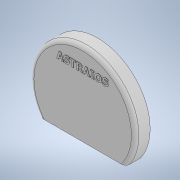
# Autodesk Inventor part: SensorCap_v2
Saved by Autodesk Inventor 2020 (Build 240168000, 168)
## iProperties
Created: 2020-03-11
Part Number: SensorCap_v2
Material: Generic
Document SubType Name: Modeling
Designer: WANG
Density: 1 g/cm^3
Appearance: Default
Author: WANG
Autodesk Inventor part; units mm, degrees
ref_plane "YZ Plane" through (0, 0, 0) normal (1, 0, 0) x (0, 1, 0)
ref_plane "XZ Plane" through (0, 0, 0) normal (0, 1, 0) x (-1, 0, 0)
ref_plane "XY Plane" through (0, 0, 0) normal (0, 0, 1) x (1, 0, 0)
sketch "Sketch1" plane through (0, 0, 0) normal (0, 0, 1) x (1, 0, 0)
  circle A0 centre (0, 0) radius 44.45
  circle A1 centre (0, 0) radius 41.275
  dimension "d0" = 88.9
  dimension "d1" = 82.55
  constraints: 2 centre point, 2 coincident
  measures "d0" diameter of A0
  measures "d1" diameter of A1
extrude "Extrusion1" add sketch "Sketch1" along normal blind 12.7 contours A0 | A1
sketch "Sketch2" plane through (0, 0, 0) normal (0, 0, -1) x (-1, 0, 0)
  circle A0 centre (0, 0) radius 44.45
  circle A1 centre (0, 0) radius 41.275
  dimension "d4" = 88.9
  dimension "d5" = 82.55
  constraints: 2 centre point, 2 coincident
  measures "d4" diameter of A0
  measures "d5" diameter of A1
extrude "Extrusion2" cut sketch "Sketch2" against normal blind 9.525 contours A1
sketch "Sketch3" plane through (0, 0, 12.7) normal (0, 0, 1) x (1, 0, 0)
  circle A0 centre (0, 0) radius 44.45
  line L0 (0, -25.4) -> (36.478, -25.4)
  line L1 (0, -25.4) -> (-36.478, -25.4)
  circle A1 centre (0, 0) radius 44.45 projected
  dimension "d8" = 88.9
  dimension "d9" = 25.4
  constraints: 4 end point, 1 coincident, 1 horizontal, 1 point on circle, 1 point on line, 3 other
  measures "d9" distance of L0.start point (0, 0)
extrude "Extrusion3" cut sketch "Sketch3" against normal up to surface (12.7 mm away) contours L1 L0 A0 picked at (-22.4742, -27.57)
fillet "Fillet1" radius 3.175 1 edges at (0, 44.45, 12.7)
sketch "Sketch4" plane through (0, 0, 12.7) normal (0, 0, 1) x (1, 0, 0)
  line L0 (-21.9003, 31.3927) -> (21.9277, 31.3927) construction
  line L1 (21.9277, 31.3927) -> (21.9277, 25.0398) construction
  line L2 (21.9277, 25.0398) -> (-21.9003, 25.0398) construction
  line L3 (-21.9003, 25.0398) -> (-21.9003, 31.3927) construction
  line L4 (-21.925, 25.1683) -> (-19.865, 31.2643)
  line L5 (-19.865, 31.2643) -> (-18.1953, 31.2643)
  line L6 (-18.1953, 31.2643) -> (-16.1353, 25.1683)
  line L7 (-16.1353, 25.1683) -> (-17.7112, 25.1683)
  line L8 (-17.7112, 25.1683) -> (-18.0915, 26.4132)
  line L9 (-18.0915, 26.4132) -> (-20.0083, 26.4132)
  line L10 (-20.0083, 26.4132) -> (-20.3936, 25.1683)
  line L11 (-20.3936, 25.1683) -> (-21.925, 25.1683)
  line L12 (-18.4275, 27.5197) -> (-19.0499, 29.5353)
  line L13 (-19.0499, 29.5353) -> (-19.6773, 27.5197)
  line L14 (-19.6773, 27.5197) -> (-18.4275, 27.5197)
  spline S0 degree 2 poles (-13.6455, 25.0596) (-14.347, 25.0596) (-15.4042, 25.3313) (-15.8587, 25.5289) knots 0 0 0 1 2 2 2
  line L15 (-15.8587, 25.5289) -> (-15.8587, 26.9813)
  line L16 (-15.8587, 26.9813) -> (-15.7203, 26.9813)
  spline S1 degree 2 poles (-15.7203, 26.9813) (-15.2609, 26.591) (-14.1593, 26.1711) (-13.6406, 26.1711) knots 0 0 0 1 2 2 2
  spline S2 degree 2 poles (-13.6406, 26.1711) (-13.5072, 26.1711) (-13.0774, 26.2304) (-12.949, 26.2897) knots 0 0 0 1 2 2 2
  spline S3 degree 2 poles (-12.949, 26.2897) (-12.7909, 26.3588) (-12.5686, 26.6108) (-12.5686, 26.8133) knots 0 0 0 1 2 2 2
  spline S4 degree 2 poles (-12.5686, 26.8133) (-12.5686, 27.0455) (-12.9292, 27.332) (-13.1762, 27.3962) knots 0 0 0 1 2 2 2
  spline S5 degree 2 poles (-13.1762, 27.3962) (-13.4874, 27.4802) (-14.1939, 27.6235) (-14.5051, 27.7321) knots 0 0 0 1 2 2 2
  spline S6 degree 2 poles (-14.5051, 27.7321) (-15.2115, 27.9791) (-15.8241, 28.8239) (-15.8241, 29.4562) knots 0 0 0 1 2 2 2
  spline S7 degree 2 poles (-15.8241, 29.4562) (-15.8241, 30.3108) (-14.3766, 31.3729) (-13.2898, 31.3729) knots 0 0 0 1 2 2 2
  spline S8 degree 2 poles (-13.2898, 31.3729) (-12.7464, 31.3729) (-11.6695, 31.1506) (-11.2447, 30.9629) knots 0 0 0 1 2 2 2
  line L17 (-11.2447, 30.9629) -> (-11.2447, 29.5698)
  line L18 (-11.2447, 29.5698) -> (-11.378, 29.5698)
  spline S9 degree 2 poles (-11.378, 29.5698) (-11.7189, 29.8613) (-12.697, 30.2614) (-13.2108, 30.2614) knots 0 0 0 1 2 2 2
  spline S10 degree 2 poles (-13.2108, 30.2614) (-13.4133, 30.2614) (-13.7295, 30.2022) (-13.9073, 30.1231) knots 0 0 0 1 2 2 2
  spline S11 degree 2 poles (-13.9073, 30.1231) (-14.0506, 30.0589) (-14.2581, 29.802) (-14.2581, 29.6439) knots 0 0 0 1 2 2 2
  spline S12 degree 2 poles (-14.2581, 29.6439) (-14.2581, 29.4068) (-13.9271, 29.1351) (-13.4529, 29.0264) knots 0 0 0 1 2 2 2
  spline S13 degree 2 poles (-13.4529, 29.0264) (-13.1466, 28.9573) (-12.5785, 28.8239) (-12.2524, 28.7103) knots 0 0 0 1 2 2 2
  spline S14 degree 2 poles (-12.2524, 28.7103) (-11.6201, 28.4781) (-11.0026, 27.7074) (-11.0026, 27.0751) knots 0 0 0 1 2 2 2
  spline S15 degree 2 poles (-11.0026, 27.0751) (-11.0026, 26.1662) (-12.4303, 25.0596) (-13.6455, 25.0596) knots 0 0 0 1 2 2 2
  line L19 (-9.0463, 25.1683) -> (-9.0463, 30.1034)
  line L20 (-9.0463, 30.1034) -> (-10.8495, 30.1034)
  line L21 (-10.8495, 30.1034) -> (-10.8495, 31.2643)
  line L22 (-10.8495, 31.2643) -> (-5.7118, 31.2643)
  line L23 (-5.7118, 31.2643) -> (-5.7118, 30.1034)
  line L24 (-5.7118, 30.1034) -> (-7.5149, 30.1034)
  line L25 (-7.5149, 30.1034) -> (-7.5149, 25.1683)
  line L26 (-7.5149, 25.1683) -> (-9.0463, 25.1683)
  line L27 (0.5472, 25.1683) -> (-1.3152, 25.1683)
  line L28 (-1.3152, 25.1683) -> (-3.0096, 27.4061)
  line L29 (-3.0096, 27.4061) -> (-3.5629, 27.4061)
  line L30 (-3.5629, 27.4061) -> (-3.5629, 25.1683)
  line L31 (-3.5629, 25.1683) -> (-5.0844, 25.1683)
  line L32 (-5.0844, 25.1683) -> (-5.0844, 31.2643)
  line L33 (-5.0844, 31.2643) -> (-2.6342, 31.2643)
  spline S16 degree 2 poles (-2.6342, 31.2643) (-2.1254, 31.2643) (-1.3745, 31.1358) (-1.0534, 30.9382) knots 0 0 0 1 2 2 2
  spline S17 degree 2 poles (-1.0534, 30.9382) (-0.7273, 30.7307) (-0.342, 30.0836) (-0.342, 29.5896) knots 0 0 0 1 2 2 2
  spline S18 degree 2 poles (-0.342, 29.5896) (-0.342, 28.893) (-0.9743, 28.0187) (-1.5029, 27.7618) knots 0 0 0 1 2 2 2
  line L34 (-1.5029, 27.7618) -> (0.5472, 25.1683)
  spline S19 degree 2 poles (-1.9129, 29.3969) (-1.9129, 29.6291) (-2.0908, 29.9601) (-2.2933, 30.049) knots 0 0 0 1 2 2 2
  spline S20 degree 2 poles (-2.2933, 30.049) (-2.4366, 30.1083) (-2.7873, 30.1429) (-3.0491, 30.1429) knots 0 0 0 1 2 2 2
  line L35 (-3.0491, 30.1429) -> (-3.5629, 30.1429)
  line L36 (-3.5629, 30.1429) -> (-3.5629, 28.5028)
  line L37 (-3.5629, 28.5028) -> (-3.1232, 28.5028)
  spline S21 degree 2 poles (-3.1232, 28.5028) (-2.8071, 28.5028) (-2.3575, 28.5818) (-2.2044, 28.7053) knots 0 0 0 1 2 2 2
  spline S22 degree 2 poles (-2.2044, 28.7053) (-2.0562, 28.8239) (-1.9129, 29.1401) (-1.9129, 29.3969) knots 0 0 0 1 2 2 2
  line L38 (0.3447, 25.1683) -> (2.4046, 31.2643)
  line L39 (2.4046, 31.2643) -> (4.0744, 31.2643)
  line L40 (4.0744, 31.2643) -> (6.1344, 25.1683)
  line L41 (6.1344, 25.1683) -> (4.5585, 25.1683)
  line L42 (4.5585, 25.1683) -> (4.1781, 26.4132)
  line L43 (4.1781, 26.4132) -> (2.2614, 26.4132)
  line L44 (2.2614, 26.4132) -> (1.8761, 25.1683)
  line L45 (1.8761, 25.1683) -> (0.3447, 25.1683)
  line L46 (3.8422, 27.5197) -> (3.2198, 29.5353)
  line L47 (3.2198, 29.5353) -> (2.5924, 27.5197)
  line L48 (2.5924, 27.5197) -> (3.8422, 27.5197)
  line L49 (9.7752, 25.1683) -> (6.495, 25.1683)
  line L50 (6.495, 25.1683) -> (6.495, 26.2304)
  line L51 (6.495, 26.2304) -> (7.3694, 26.2304)
  line L52 (7.3694, 26.2304) -> (7.3694, 30.2022)
  line L53 (7.3694, 30.2022) -> (6.495, 30.2022)
  line L54 (6.495, 30.2022) -> (6.495, 31.2643)
  line L55 (6.495, 31.2643) -> (9.7752, 31.2643)
  line L56 (9.7752, 31.2643) -> (9.7752, 30.2022)
  line L57 (9.7752, 30.2022) -> (8.9008, 30.2022)
  line L58 (8.9008, 30.2022) -> (8.9008, 26.2304)
  line L59 (8.9008, 26.2304) -> (9.7752, 26.2304)
  line L60 (9.7752, 26.2304) -> (9.7752, 25.1683)
  spline S23 degree 2 poles (16.3405, 28.2163) (16.3405, 26.7343) (14.7597, 25.0398) (13.3863, 25.0398) knots 0 0 0 1 2 2 2
  spline S24 degree 2 poles (13.3863, 25.0398) (12.0081, 25.0398) (10.4371, 26.754) (10.4371, 28.2163) knots 0 0 0 1 2 2 2
  spline S25 degree 2 poles (10.4371, 28.2163) (10.4371, 29.6835) (12.0081, 31.3927) (13.3863, 31.3927) knots 0 0 0 1 2 2 2
  spline S26 degree 2 poles (13.3863, 31.3927) (14.7597, 31.3927) (16.3405, 29.6933) (16.3405, 28.2163) knots 0 0 0 1 2 2 2
  spline S27 degree 2 poles (14.7597, 28.2163) (14.7597, 28.7646) (14.5374, 29.5303) (14.3447, 29.7724) knots 0 0 0 1 2 2 2
  spline S28 degree 2 poles (14.3447, 29.7724) (14.152, 30.0243) (13.658, 30.2417) (13.3913, 30.2417) knots 0 0 0 1 2 2 2
  spline S29 degree 2 poles (13.3913, 30.2417) (13.1097, 30.2417) (12.6503, 30.0391) (12.4379, 29.7823) knots 0 0 0 1 2 2 2
  spline S30 degree 2 poles (12.4379, 29.7823) (12.2501, 29.5451) (12.018, 28.7597) (12.018, 28.2163) knots 0 0 0 1 2 2 2
  spline S31 degree 2 poles (12.018, 28.2163) (12.018, 27.6531) (12.2403, 26.9121) (12.4329, 26.6602) knots 0 0 0 1 2 2 2
  spline S32 degree 2 poles (12.4329, 26.6602) (12.6256, 26.4082) (13.1245, 26.1909) (13.3913, 26.1909) knots 0 0 0 1 2 2 2
  spline S33 degree 2 poles (13.3913, 26.1909) (13.663, 26.1909) (14.1669, 26.423) (14.3496, 26.67) knots 0 0 0 1 2 2 2
  spline S34 degree 2 poles (14.3496, 26.67) (14.5472, 26.9368) (14.7597, 27.6432) (14.7597, 28.2163) knots 0 0 0 1 2 2 2
  spline S35 degree 2 poles (19.1316, 25.0596) (18.4301, 25.0596) (17.3729, 25.3313) (16.9185, 25.5289) knots 0 0 0 1 2 2 2
  line L61 (16.9185, 25.5289) -> (16.9185, 26.9813)
  line L62 (16.9185, 26.9813) -> (17.0568, 26.9813)
  spline S36 degree 2 poles (17.0568, 26.9813) (17.5162, 26.591) (18.6178, 26.1711) (19.1365, 26.1711) knots 0 0 0 1 2 2 2
  spline S37 degree 2 poles (19.1365, 26.1711) (19.2699, 26.1711) (19.6997, 26.2304) (19.8281, 26.2897) knots 0 0 0 1 2 2 2
  spline S38 degree 2 poles (19.8281, 26.2897) (19.9862, 26.3588) (20.2085, 26.6108) (20.2085, 26.8133) knots 0 0 0 1 2 2 2
  spline S39 degree 2 poles (20.2085, 26.8133) (20.2085, 27.0455) (19.8479, 27.332) (19.6009, 27.3962) knots 0 0 0 1 2 2 2
  spline S40 degree 2 poles (19.6009, 27.3962) (19.2897, 27.4802) (18.5833, 27.6235) (18.272, 27.7321) knots 0 0 0 1 2 2 2
  spline S41 degree 2 poles (18.272, 27.7321) (17.5656, 27.9791) (16.953, 28.8239) (16.953, 29.4562) knots 0 0 0 1 2 2 2
  spline S42 degree 2 poles (16.953, 29.4562) (16.953, 30.3108) (18.4005, 31.3729) (19.4873, 31.3729) knots 0 0 0 1 2 2 2
  spline S43 degree 2 poles (19.4873, 31.3729) (20.0307, 31.3729) (21.1076, 31.1506) (21.5325, 30.9629) knots 0 0 0 1 2 2 2
  line L63 (21.5325, 30.9629) -> (21.5325, 29.5698)
  line L64 (21.5325, 29.5698) -> (21.3991, 29.5698)
  spline S44 degree 2 poles (21.3991, 29.5698) (21.0582, 29.8613) (20.0801, 30.2614) (19.5663, 30.2614) knots 0 0 0 1 2 2 2
  spline S45 degree 2 poles (19.5663, 30.2614) (19.3638, 30.2614) (19.0476, 30.2022) (18.8698, 30.1231) knots 0 0 0 1 2 2 2
  spline S46 degree 2 poles (18.8698, 30.1231) (18.7265, 30.0589) (18.519, 29.802) (18.519, 29.6439) knots 0 0 0 1 2 2 2
  spline S47 degree 2 poles (18.519, 29.6439) (18.519, 29.4068) (18.85, 29.1351) (19.3243, 29.0264) knots 0 0 0 1 2 2 2
  spline S48 degree 2 poles (19.3243, 29.0264) (19.6305, 28.9573) (20.1986, 28.8239) (20.5247, 28.7103) knots 0 0 0 1 2 2 2
  spline S49 degree 2 poles (20.5247, 28.7103) (21.157, 28.4781) (21.7745, 27.7074) (21.7745, 27.0751) knots 0 0 0 1 2 2 2
  spline S50 degree 2 poles (21.7745, 27.0751) (21.7745, 26.1662) (20.3468, 25.0596) (19.1316, 25.0596) knots 0 0 0 1 2 2 2
  point P0 (0, 0)
  constraints: 2 other
emboss "Emboss1" sketch "Sketch4" operation add depth 0.254 direction (0, 0, -1)
body "Solid1"
